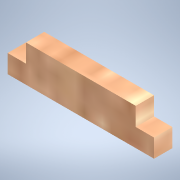
# Autodesk Inventor part: beam1
Saved by Autodesk Inventor 2022 (Build 260153000, 153)
## iProperties
Created: 2021-12-11
Part Number: beam1
Material: Wood (Birch)
Document SubType Name: Modeling
Designer: dangl
Density: 0.55 g/cm^3
Appearance: Birch - Natural Polished
Author: dangl
Autodesk Inventor part; units mm, degrees
ref_plane "YZ Plane" through (0, 0, 0) normal (1, 0, 0) x (0, 1, 0)
ref_plane "XZ Plane" through (0, 0, 0) normal (0, 1, 0) x (-1, 0, 0)
ref_plane "XY Plane" through (0, 0, 0) normal (0, 0, 1) x (1, 0, 0)
sketch "Sketch1" plane through (0, 0, 0) normal (0, 0, 1) x (1, 0, 0)
  line L0 (0, 0) -> (-50, 0)
  line L1 (-50, 0) -> (-50, 2)
  line L2 (-46, 4) -> (-46, 2)
  line L3 (-46, 2) -> (-50, 2)
  line L4 (0, 2) -> (-4, 2)
  line L5 (-4, 2) -> (-4, 4)
  line L6 (-46, 4) -> (-26, 4)
  line L7 (0, 2) -> (0, 0)
  line L8 (-26, 4) -> (-26, 2)
  line L9 (-26, 2) -> (-24, 2)
  line L10 (-24, 2) -> (-24, 4)
  line L11 (-24, 4) -> (-4, 4)
  dimension "d2" = 4
  dimension "d3" = 2
  dimension "d5" = 24
  dimension "d6" = 2
  dimension "d7" = 2
  constraints: 24 end point, 4 parallel, 2 horizontal, 2 perpendicular, 1 point on line
  measures "d2" distance of L2.end L1.end
  measures "d3" distance of L2.start L2.end
  measures "d5" distance from line of L0.start L10
  measures "d6" distance of L8.end L9.end
  measures "d7" distance of L9.end L10.end
extrude "Extrusion1" add sketch "Sketch1" along normal blind 2
sketch "Sketch2" plane through (0, 0, 2) normal (0, 0, 1) x (1, 0, 0)
  line L0 (-4, 4) -> (-24, 4) projected
  line L1 (-18, 4) -> (-16, 4)
  line L2 (-16, 4) -> (-16, 2)
  line L3 (-16, 2) -> (-18, 2)
  line L4 (-18, 2) -> (-18, 4)
  point P0 (0, 0)
  dimension "d10" = 2
  dimension "d11" = 2
  dimension "d12" = 16
  constraints: 8 end point, 2 parallel, 1 horizontal, 1 perpendicular, 1 point on line
  measures "d10" distance of L2.end L3.end
  measures "d11" distance of L1.end L2.end
  measures "d12" distance from line of point (0, 0) L2
extrude "Extrusion2" cut sketch "Sketch2" against normal blind 2
sketch "Sketch3" plane through (0, 0, 0) normal (0, 0, -1) x (-1, 0, 0)
  line L0 (18, 4) -> (24, 4) projected
  line L1 (50, 2) -> (50, 0) projected
  line L2 (18, 4) -> (50, 4)
  line L3 (50, 4) -> (50, 0)
  line L4 (50, 0) -> (18, 0)
  line L5 (18, 0) -> (18, 4)
  line L6 (0, 2) -> (4, 2) projected
  line L7 (0, 0) -> (0, 2) projected
  line L8 (4, 2) -> (0, 2)
  line L9 (0, 2) -> (0, 0)
  line L10 (0, 0) -> (4, 0)
  line L11 (4, 0) -> (4, 2)
  line L12 (4, 2) -> (4, 4) projected
  line L13 (4, 4) -> (6, 4)
  line L14 (6, 4) -> (6, 2)
  line L15 (6, 2) -> (4, 2)
  line L16 (4, 2) -> (4, 4)
  dimension "d17" = 2
  constraints: 24 end point, 6 parallel, 3 horizontal, 3 perpendicular, 1 point on line
  measures "d17" distance of L14.end L15.end
extrude "Extrusion3" cut sketch "Sketch3" against normal blind 10
body "Solid1"
